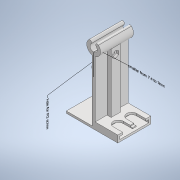
# Autodesk Inventor part: prototype7_1
Saved by Autodesk Inventor 2022 (Build 260153000, 153)
## iProperties
Created: 2022-06-15
Part Number: prototype7_1
Material: Generic
Document SubType Name: Modeling
Designer: tecware
Density: 1 g/cm^3
Appearance: Default
Author: tecware
## iProperties of the stored document prototype_8_1_3DPrint.ipt
Created: 2022-06-16
Part Number: prototype_8_1_3DPrint
Material: Generic
Document SubType Name: Modeling
Designer: tecware
Density: 1 g/cm^3
Appearance: Default
Author: tecware
Autodesk Inventor part; units mm, degrees
ref_plane "YZ Plane" through (0, 0, 0) normal (1, 0, 0) x (0, 1, 0)
ref_plane "XZ Plane" through (0, 0, 0) normal (0, 1, 0) x (-1, 0, 0)
ref_plane "XY Plane" through (0, 0, 0) normal (0, 0, 1) x (1, 0, 0)
sketch "Sketch1" plane through (0, 0, 0) normal (0, 1, 0) x (-1, 0, 0)
  line L0 (11, -16) -> (-11, -16)
  line L1 (-11, -16) -> (-11, 16)
  line L2 (-11, 16) -> (11, 16)
  line L3 (11, 16) -> (11, -16)
  line L4 (11, -16) -> (-11, 16) construction
  line L5 (-11, -16) -> (11, 16) construction
  circle A0 centre (-2, 6.5) radius 4.8
  line L6 (-2, 6.5) -> (-2, -6.5)
  circle A1 centre (-2, -6.5) radius 4.8
  line L7 (-2, 11.3) -> (-11, 11.3)
  line L8 (-2, 1.7) -> (-11, 1.7)
  line L9 (-2, -1.7) -> (-11, -1.7)
  line L10 (-2, -11.3) -> (-11, -11.3)
  point P0 (0, 0)
  point P1 (-2, 0)
  dimension "d0" = 22
  dimension "d1" = 32
  dimension "d2" = 9.6
  dimension "d3" = 13
  dimension "d4" = 9.6
  constraints: 22 end point, 6 point on line, 4 point on circle, 3 midpoint, 2 centre point, 2 perpendicular, 1 coincident, 1 horizontal, 1 vertical
  measures "d0" distance of L1.end L2.end
  measures "d1" distance of L0.end L1.end
  measures "d2" diameter of A0
  measures "d3" distance of L6.start L6.end
  measures "d4" diameter of A1
extrude "Extrusion1" add sketch "Sketch1" along normal blind 2 contours L0 L1 L10 A1 L6 A0 L7 L2 L3 | L1 L8 L6 L9
sketch "Sketch2" plane through (0, 0, 0) normal (0, -1, 0) x (1, 0, 0)
  line L0 (-11, 16) -> (11, 16) projected
  line L1 (11, 16) -> (-11, 16)
  line L2 (-11, -16) -> (-11, 16) projected
  line L3 (-11, 16) -> (-11, -16)
  line L4 (11, -16) -> (-11, -16) projected
  line L5 (-11, -16) -> (11, -16)
  line L6 (11, -16) -> (11, -14)
  line L7 (11, -11.3) -> (11, -16) projected
  line L8 (11, -14) -> (-5, -14)
  line L9 (-5, -14) -> (-5, 14)
  line L10 (-5, 14) -> (11, 14)
  line L11 (11, 16) -> (11, 11.3) projected
  point P0 (0, 0)
  dimension "d7" = 2
  dimension "d8" = 16
  dimension "d9" = 28
  constraints: 14 end point, 2 point on line
  measures "d7" distance of L4.start L6.end
  measures "d8" distance of L6.end L8.end
  measures "d9" distance of L8.end L9.end
extrude "Extrusion2" add sketch "Sketch2" along normal blind 2.75
sketch "Sketch3" plane through (-11, 2, -16) normal (-1, 0, 0) x (0, 0, 1)
  line L0 (0, 0) -> (0, -4.75) projected
  line L1 (0, -4.75) -> (32, -4.75)
  line L2 (32, -4.75) -> (32, 49.75)
  line L3 (32, 49.75) -> (0, 49.75)
  line L4 (0, 49.75) -> (0, -4.75)
  point P0 (16, -2)
  dimension "d12" = 54.5
  constraints: 8 end point
  measures "d12" distance of L2.end L1.end
extrude "Extrusion3" add sketch "Sketch3" along normal blind 3
sketch "Sketch4" plane through (0, -2.75, 0) normal (0, -1, 0) x (1, 0, 0)
  line L0 (11, 16) -> (11, 11.3) projected
  line L1 (11, 16) -> (-39, 16)
  line L2 (-39, 16) -> (-39, -16)
  line L3 (-39, -16) -> (11, -16)
  line L4 (11, -16) -> (11, 16)
  point P0 (0, 0)
  dimension "d15" = 50
  constraints: 8 end point
  measures "d15" distance of L3.end L2.end
extrude "Extrusion4" add sketch "Sketch4" along normal blind 2
sketch "Sketch5" plane through (-5, 0, 14) normal (1, 0, 0) x (0, 0, -1)
  line L0 (0, 0) -> (0, -2.75) projected
  line L1 (30, -2.75) -> (-2, -2.75) projected
  line L2 (0, 0) -> (2.9896, 0)
  line L3 (2.9896, 0) -> (2.9896, -2.75)
  line L4 (2.9896, -2.75) -> (0, -2.5)
  line L5 (0, -2.5) -> (0, 0)
  point P0 (14, 0)
  dimension "d18" = 3
  constraints: 8 end point, 1 point on line
  measures "d18" distance of L3.end L4.end
extrude "Extrusion5" cut sketch "Sketch5" against normal up to surface (9 mm away)
sketch "Sketch6" plane through (11, 0, 1.7) normal (1, 0, 0) x (0, 0, -1)
  line L0 (0, 0) -> (0, 2) projected
  line L1 (3.4, 0) -> (3.4, 2) projected
  line L2 (0, 1) -> (3.4, 1)
  line L3 (3.4, 1) -> (3.4, 2)
  line L4 (3.4, 2) -> (0, 2)
  line L5 (0, 2) -> (0, 1)
  point P0 (1.7, 0)
  constraints: 8 end point, 1 midpoint
extrude "Extrusion6" cut sketch "Sketch6" against normal blind 2.2
sketch "Sketch8" plane through (-14, 2, -16) normal (-1, 0, 0) x (0, 0, 1)
  circle A0 centre (24.6, 39.75) radius 2.75
  circle A1 centre (24.6, 39.75) radius 1.4
  line L0 (4, 47.25) -> (28, 47.25) construction
  line L1 (28, 47.25) -> (28, -1.75) construction
  line L2 (28, -1.75) -> (4, -1.75) construction
  line L3 (4, -1.75) -> (4, 47.25) construction
  circle A2 centre (7.4, 5.75) radius 2.75
  circle A3 centre (7.4, 5.75) radius 1.4
  line L4 (4, 47.25) -> (28, -1.75) construction
  line L5 (32, -4.75) -> (32, -6.75) construction
  line L6 (32, 49.75) -> (0, 49.75) construction
  line L7 (0, -4.75) -> (32, 49.75) construction
  point P0 (16, -2)
  point P1 (16, 22.75)
  point P2 (16, 22.5)
  dimension "d24" = 5.5
  dimension "d25" = 2.8
  dimension "d26" = 24
  dimension "d27" = 49
  dimension "d28" = 3.4
  dimension "d29" = 7.5
  dimension "d30" = 5.5
  dimension "d31" = 2.8
  dimension "d32" = 3.4
  dimension "d33" = 7.5
  constraints: 12 end point, 4 centre point, 2 coincident, 2 midpoint
  measures "d24" diameter of A0
  measures "d25" diameter of A1
  measures "d26" distance of L1.end L2.end
  measures "d27" distance of L0.end L1.end
  measures "d28" distance from line of L1 A0.centre
  measures "d29" distance from line of L0 A0.centre
  measures "d30" diameter of A2
  measures "d31" diameter of A3
  measures "d32" distance from line of L3 A3.centre
  measures "d33" distance from line of L2 A3.centre
extrude "Extrusion7" add sketch "Sketch8" along normal blind 5
sketch "Sketch9" plane through (0, 0, 0) normal (0, 0, 1) x (1, 0, 0)
  line L0 (-14, -2.75) -> (-14, 51.75) projected
  line L1 (-12.5, 56.75) -> (-12.5, 54.25) construction
  line L2 (-12.25, 56.75) -> (-12.25, 54.25)
  line L3 (-12.25, 54.25) -> (-12.75, 54.25)
  line L4 (-12.75, 54.25) -> (-12.75, 56.75)
  line L5 (-12.75, 56.75) -> (-12.25, 54.25) construction
  line L6 (-12.25, 56.75) -> (-12.75, 54.25) construction
  circle A0 centre (-12.5, 63.45) radius 6.7
  line L7 (-12.5, 63.45) -> (-12.5, 56.75) construction
  line L8 (-12.25, 56.75) -> (-12.25, 59.7585)
  line L9 (-12.75, 59.7585) -> (-12.75, 56.75)
  line L10 (-12.25, 59.7585) -> (-12.25, 70.1453)
  line L11 (-12.25, 70.1453) -> (-12.75, 70.1453)
  line L12 (-12.75, 70.1453) -> (-12.75, 59.7585)
  line L13 (-12.5, 63.45) -> (-5.8, 63.45) construction
  line L14 (-12.5, 63.45) -> (-5.8, 63.45) construction
  line L15 (-11, 51.75) -> (-14, 51.75) projected
  line L16 (-14, 51.75) -> (-11, 51.75)
  line L17 (-11, 51.75) -> (-11, 56.75)
  line L18 (-11, 56.75) -> (-14, 56.75)
  line L19 (-14, 56.75) -> (-14, 51.75)
  line L20 (-14, 56.75) -> (-11, 56.75)
  line L21 (-11, 56.75) -> (-11, 56.9201)
  line L22 (-11, 56.9201) -> (-14, 56.9201)
  line L23 (-14, 56.9201) -> (-14, 56.75)
  circle A1 centre (-12.5, 63.45) radius 3.5
  line L24 (-12.5, 63.45) -> (-5.8, 63.45) construction
  line L25 (-12.5, 63.45) -> (-5.8, 63.45) construction
  circle A2 centre (-16.1062, 67.0562) radius 1.6
  circle A3 centre (-8.8938, 67.0562) radius 1.6
  point P0 (0, 0)
  point P1 (-12.5, 55.5)
  point P2 (-12.75, 56.7547)
  point P3 (-12.25, 56.7547)
  point P4 (-17.2376, 68.1876)
  point P5 (-12.75, 59.9589)
  point P6 (-14.9749, 65.9249)
  point P7 (-10.0251, 65.9249)
  point P8 (-12.25, 59.9589)
  point P9 (-7.7624, 68.1876)
  dimension "d47" = 0.5
  dimension "d49" = 13.4
  dimension "d50" = 5
  dimension "d57" = 7
  constraints: 48 end point, 4 centre point, 4 horizontal, 3 midpoint, 3 point on circle, 1 point on line
  measures "d47" distance of L3.start L3.end
  measures "d49" diameter of A0
  measures "d50" distance of L17.end L16.end
  measures "d57" diameter of A1
extrude "Extrusion8" add sketch "Sketch9" along normal mid plane 32 contours L18 L17 L15 L19 L4 L3 L2 | L8 A0 L21 L18 | L8 L22 A0 | L22 L8 L10 A1 A3 A0 | L9 L18 L23 A0 | A0 L22 L9 | L22 A0 A2 A1 L12 L9 | A3 | A2
sketch "Sketch10" plane through (-11, 2, 16) normal (0, 0, 1) x (1, 0, 0)
  line L0 (-1.75, 52.25) -> (-1.25, 52.25) projected
  line L1 (-1.75, 52.25) -> (-1.25, 52.25)
  line L2 (-1.25, 52.25) -> (-1.25, 37.25)
  line L3 (-1.25, 37.25) -> (-1.75, 37.25)
  line L4 (-1.75, 37.25) -> (-1.75, 52.25)
  line L5 (-1.75, 37.25) -> (-2.4777, 58.0893)
  arc A0 (-3.9749, 63.9249) -> (-1.75, 57.9589) centre (-1.5, 61.45) ccw projected
  line L6 (-1.75, 37.25) -> (19.102, 37.25) construction
  line L7 (-1.25, 37.25) -> (-0.5223, 58.0893)
  arc A1 (-1.25, 57.9589) -> (0.9749, 63.9249) centre (-1.5, 61.45) ccw projected
  line L8 (-1.25, 37.25) -> (19.602, 37.25) construction
  arc A2 (-2.4777, 58.0893) -> (-0.5223, 58.0893) centre (-1.5, 61.45) ccw
  point P0 (11, -2)
  dimension "d51" = 15
  dimension "d60" = 92
  dimension "d61" = 88
  constraints: 16 end point, 4 point on circle, 2 equal length, 2 horizontal, 1 centre point
  measures "d51" distance of L1.end L2.end
  measures "d60" angle of L6 L5
  measures "d61" angle of L8 L7
extrude "Extrusion9" cut sketch "Sketch10" against normal through all contours L0 L2 L3 L4
sketch "Sketch11" plane through (0, 0, 0) normal (0, 0, 1) x (1, 0, 0)
  line L0 (-14, -2.75) -> (-14, 56.9201) projected
  line L1 (-12.5, 63.45) -> (-18.3024, 60.1)
  line L2 (-14, 56.9201) -> (-14, 62.9804)
  circle A0 centre (-12.5, 63.45) radius 6.7
  point P0 (0, 0)
  point P1 (-14, 62.584)
  constraints: 4 end point, 2 coincident, 3 other
extrude "Extrusion10" cut sketch "Sketch11" along normal mid plane 10 contours L2 A0 L1 picked at (-14.4333, 58.9557)
sketch "Sketch13" plane through (0, 2, 0) normal (0, 1, 0) x (1, 0, 0)
  line L0 (-11, 16) -> (-11, -16) projected
  line L1 (-11, 0) -> (-9, 0) construction
  line L2 (-11, 4.5) -> (-7, 4.5)
  line L3 (-7, 4.5) -> (-7, -4.5)
  line L4 (-7, -4.5) -> (-11, -4.5)
  line L5 (-11, -4.5) -> (-11, 4.5)
  line L6 (-11, 4.5) -> (-7, -4.5) construction
  line L7 (-7, 4.5) -> (-11, -4.5) construction
  point P0 (0, 0)
  point P1 (-11, -4.5)
  dimension "d66" = 2
  dimension "d67" = 4
  dimension "d68" = 9
  constraints: 14 end point, 3 midpoint, 3 perpendicular
  measures "d66" distance of L1.start L1.end
  measures "d67" distance of L3.end L4.end
  measures "d68" distance of L2.end L3.end
extrude "Extrusion12" add sketch "Sketch13" along normal up to surface round surface about axis through (-12.5, 63.45, 0) along (0, 0, 1) radius 6.7 far side no
sketch "Sketch12" plane through (-14, 2, -16) normal (-1, 0, 0) x (0, 0, 1)
  line L0 (0, 54.9201) -> (32, 54.9201) projected
  line L1 (16, 54.9201) -> (16, 50.9201) construction
  circle A0 centre (16, 50.9201) radius 1.5
  point P0 (16, -2)
  dimension "d62" = 4
  dimension "d63" = 3
  constraints: 2 end point, 1 centre point, 1 coincident, 1 midpoint
  measures "d62" distance of L1.start L1.end
  measures "d63" diameter of A0
extrude "Extrusion11" cut sketch "Sketch12" against normal through all
sketch "Sketch14" plane through (-7, 2, 4.5) normal (1, 0, 0) x (0, 0, -1)
  line L0 (7.4, 49.2458) -> (4.5, 47.5714)
  line L1 (4.5, 47.5714) -> (1.6, 49.2458)
  line L2 (1.6, 49.2458) -> (1.6, 52.5944)
  line L3 (1.6, 52.5944) -> (4.5, 54.2687)
  line L4 (4.5, 54.2687) -> (7.4, 52.5944)
  line L5 (7.4, 52.5944) -> (7.4, 49.2458)
  circle A0 centre (4.5, 50.9201) radius 1.5 projected
  point P0 (4.5, -2)
  point P1 (4.5, 50.9201)
  dimension "d71" = 5.8
  dimension "d74" = 0
  constraints: 12 end point, 1 coincident, 1 vertical, 13 other
  measures "d71" distance between parallel lines of L5 L2
  measures "d74" distance of A0.centre point (4.5, 50.92)
extrude "Extrusion13" cut sketch "Sketch14" against normal blind 2.5
body "Solid1"
